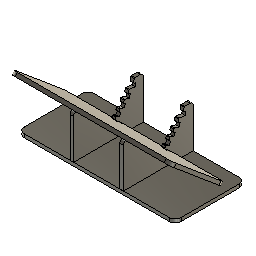
Stand1 (Autodesk Fusion 360 design; units mm, degrees)
Autodesk Fusion 360 part; units mm, degrees
sketch "スケッチ1" plane through (0, 0, 0) normal (0, 0, 1) x (1, 0, 0) in component "top1"
  line L0 (0, 0) -> (138, 0)
  line L1 (138, 0) -> (138, 60)
  line L2 (138, 60) -> (0, 60)
  line L3 (0, 60) -> (0, 0)
  line L4 (46.1, 60) -> (49, 60)
  line L5 (49, 60) -> (49, 54)
  line L6 (49, 54) -> (46.1, 54)
  line L7 (46.1, 54) -> (46.1, 60)
  line L8 (89, 60) -> (91.9, 60)
  line L9 (91.9, 60) -> (91.9, 54)
  line L10 (91.9, 54) -> (89, 54)
  line L11 (89, 54) -> (89, 60)
  line L12 (0, 60) -> (46.1, 54) construction
  line L13 (91.9, 54) -> (138, 60) construction
  line L14 (49, 54) -> (89, 54) construction
  dimension "d1" = 138
  dimension "d2" = 60
  dimension "d52" = 2.9
  dimension "d53" = 6
  dimension "d54" = 40
  constraint horizontal L0
  constraint vertical L1
  constraint horizontal L2
  constraint vertical L3
  constraint coincident L0.start L3.end
  constraint horizontal L4
  constraint vertical L5
  constraint horizontal L6
  constraint vertical L7
  constraint coincident L2 L4.start
  constraint horizontal L8
  constraint vertical L9
  constraint horizontal L10
  constraint vertical L11
  constraint coincident L2 L8.start
  constraint equal L5 L11
  constraint equal L6 L10
  constraint equal L12 L13
  measures "d1" distance of L0.start L0.end
  measures "d2" distance of L0.start L2.end
  measures "d52" distance of L5.end L6.end
  measures "d53" distance of L4.start L6.end
  measures "d54" distance of L5.end L10.end
extrude "押し出し1" add sketch "スケッチ1" along normal blind 3 contours L0 L1 L2 L3 L5 L6 L7 L9 L10 L11 makes body 1 in component "top1"
sketch "スケッチ1 (2)" plane through (0, 0, 0) normal (0, 0, 1) x (1, 0, 0) in component "base1"
  line L0 (-154.8575, 0.2102) -> (-19.8575, 0.2102)
  line L1 (-19.8575, 0.2102) -> (-19.8575, 60.2102)
  line L2 (-19.8575, 60.2102) -> (-154.8575, 60.2102)
  line L3 (-154.8575, 60.2102) -> (-154.8575, 0.2102)
  line L4 (-110.2575, 35.2102) -> (-107.3575, 35.2102)
  line L5 (-107.3575, 35.2102) -> (-107.3575, 25.2102)
  line L6 (-107.3575, 25.2102) -> (-110.2575, 25.2102)
  line L7 (-110.2575, 25.2102) -> (-110.2575, 35.2102)
  line L8 (-67.3575, 35.2102) -> (-64.4575, 35.2102)
  line L9 (-64.4575, 35.2102) -> (-64.4575, 25.2102)
  line L10 (-64.4575, 25.2102) -> (-67.3575, 25.2102)
  line L11 (-67.3575, 25.2102) -> (-67.3575, 35.2102)
  line L12 (-110.2575, 30.2102) -> (-154.8575, 30.2102) construction
  line L13 (-64.4575, 30.2102) -> (-19.8575, 30.2102) construction
  line L14 (-107.3575, 30.2102) -> (-67.3575, 30.2102) construction
  dimension "d5" = 135
  dimension "d6" = 60
  dimension "d45" = 10
  dimension "d46" = 2.9
  dimension "d47" = 40
  constraint horizontal L0
  constraint vertical L1
  constraint horizontal L2
  constraint vertical L3
  constraint horizontal L4
  constraint vertical L5
  constraint horizontal L6
  constraint vertical L7
  constraint horizontal L8
  constraint vertical L9
  constraint horizontal L10
  constraint vertical L11
  constraint equal L5 L11
  constraint equal L4 L8
  constraint midpoint L7 L12.start
  constraint midpoint L3 L12.end
  constraint midpoint L9 L13.start
  constraint midpoint L1 L13.end
  constraint midpoint L5 L14.start
  constraint midpoint L11 L14.end
  constraint horizontal L12
  constraint horizontal L14
  constraint equal L12 L13
  measures "d5" distance of L0.start L0.end
  measures "d6" distance of L0.start L2.end
  measures "d45" distance of L4.start L6.end
  measures "d46" distance of L4.start L4.end
  measures "d47" distance of L14.start L14.end
extrude "押し出し1'" add sketch "スケッチ1 (2)" along normal blind 3 separate body makes body 2 in component "base1"
sketch "スケッチ1 (3)" plane through (0, 0, 0) normal (1, 0, 0) x (0, 1, 0) in component "leg1"
  line L0 (82.5839, 7.0167) -> (142.5839, 7.0167)
  line L1 (142.5839, 7.0167) -> (142.5839, 43.8195)
  line L2 (142.5839, 43.8195) -> (82.5839, 43.8195)
  line L3 (82.5839, 43.8195) -> (82.5839, 7.0167)
  line L4 (116.2681, 18.4163) -> (82.5839, 46.6808)
  line L5 (107.5839, 7.0167) -> (117.5839, 7.0167)
  line L6 (117.5839, 7.0167) -> (117.5839, 4.1167)
  line L7 (117.5839, 4.1167) -> (107.5839, 4.1167)
  line L8 (107.5839, 4.1167) -> (107.5839, 7.0167)
  line L9 (112.5839, 4.1167) -> (112.5839, 7.0167) construction
  line L10 (83.1719, 45.4622) -> (119.7719, 22.592) construction
  line L11 (116.2681, 18.4163) -> (117.8002, 17.1308)
  line L12 (117.8002, 17.1308) -> (119.7286, 19.4289)
  line L13 (119.7286, 19.4289) -> (118.1965, 20.7145)
  line L14 (83.1268, 44.9274) -> (123.4494, 26.9747) construction
  line L15 (119.7719, 22.592) -> (121.8255, 21.3087)
  line L16 (121.8255, 21.3087) -> (123.4153, 23.8529)
  line L17 (123.4153, 23.8529) -> (121.7192, 24.9127)
  line L18 (82.9195, 44.5409) -> (127.47, 31.7662) construction
  line L19 (123.4494, 26.9747) -> (126.0624, 25.8113)
  line L20 (126.0624, 25.8113) -> (127.2826, 28.5519)
  line L21 (127.2826, 28.5519) -> (125.4555, 29.3654)
  line L22 (127.47, 31.7662) -> (130.6765, 30.8468)
  line L23 (116.2681, 18.4163) -> (137.5839, 43.8195)
  line L24 (82.5839, 44.1954) -> (132.0642, 37.2414) construction
  line L25 (132.0642, 37.2414) -> (135.9011, 36.7022)
  line L26 (135.9011, 36.7022) -> (136.3186, 39.673)
  line L27 (136.3186, 39.673) -> (134.3381, 39.9513)
  circle A0 centre (85.0839, 41.3195) radius 2.5
  line L28 (118.1965, 20.7145) -> (119.4826, 22.7727)
  line L29 (121.7192, 24.9127) -> (122.7716, 27.2764)
  line L30 (122.7716, 27.2764) -> (123.4494, 26.9747)
  line L31 (125.4555, 29.3654) -> (126.2447, 32.1176)
  line L32 (126.2447, 32.1176) -> (127.47, 31.7662)
  line L33 (130.146, 37.511) -> (132.0642, 37.2414)
  line L34 (134.3381, 39.9513) -> (134.8818, 43.8195)
  line L35 (119.4826, 22.7727) -> (119.7719, 22.592)
  line L36 (130.6765, 30.8468) -> (131.5034, 33.7306)
  line L37 (131.5034, 33.7306) -> (129.5809, 34.2818)
  line L38 (129.5809, 34.2818) -> (130.146, 37.511)
  dimension "d16" = 10
  dimension "d17" = 2.9
  dimension "d26" = 3
  dimension "d27" = 8
  dimension "d28" = 8
  dimension "d29" = 8
  dimension "d36" = 2
  dimension "d40" = 60
  dimension "d41" = 5
  dimension "d63" = 8
  dimension "d68" = 5
  dimension "d81" = 8
  constraint horizontal L0
  constraint vertical L1
  constraint horizontal L2
  constraint vertical L3
  constraint coincident L3 L24.start
  constraint horizontal L5
  constraint vertical L6
  constraint horizontal L7
  constraint vertical L8
  constraint coincident L0 L5.start
  constraint midpoint L7 L9.start
  constraint midpoint L0 L9.end
  constraint vertical L9
  constraint perpendicular L11 L12
  constraint perpendicular L10 L16
  constraint collinear L10 L15
  constraint equal L12 L16
  constraint perpendicular L19 L20
  constraint perpendicular L20 L21
  constraint collinear L14 L19
  constraint collinear L18 L22
  constraint equal L16 L20
  constraint coincident L10.end L23
  constraint coincident L13.end L23
  constraint coincident L17.end L23
  constraint coincident L14.end L23
  constraint coincident L21.end L23
  constraint coincident L18.end L23
  constraint equal L13 L17
  constraint equal L17 L21
  constraint perpendicular L4 L23
  constraint coincident L23.end L2
  constraint coincident L23 L24.end
  constraint perpendicular L25 L26
  constraint coincident L23 L27.end
  constraint perpendicular L26 L27
  constraint collinear L24 L25
  constraint collinear L4 L11
  constraint perpendicular L12 L13
  constraint perpendicular L16 L17
  constraint tangent L3 A0
  constraint tangent L2 A0
  constraint coincident L3 L4.end
  constraint tangent L4 A0
  constraint tangent L10 A0
  constraint tangent L14 A0
  constraint tangent L18 A0
  constraint tangent L24 A0
  constraint coincident L10 L28.end
  constraint perpendicular L10 L28
  constraint coincident L14 L29.end
  constraint perpendicular L14 L29
  constraint coincident L18 L31.end
  constraint perpendicular L18 L31
  constraint coincident L24 L33.start
  constraint coincident L2 L34.end
  constraint perpendicular L27 L34
  constraint perpendicular L22 L36
  constraint coincident L23 L37.end
  constraint perpendicular L36 L37
  constraint equal L20 L36
  constraint equal L26 L36
  constraint equal L21 L37
  constraint equal L27 L37
  measures "d16" distance of L5.start L5.end
  measures "d17" distance of L5.start L7.end
  measures "d26" distance of L11.end L12.end
  measures "d27" angle of L4 L10
  measures "d28" angle of L10 L14
  measures "d29" angle of L14 L18
  measures "d36" distance of L12.end L13.end
  measures "d40" distance of L0.start L0.end
  measures "d41" distance of L23.end L1.end
  measures "d63" angle of L2 L24
  measures "d68" diameter of A0
  measures "d81" angle of L18 L24
extrude "押し出し1''" add sketch "スケッチ1 (3)" along normal blind 3 separate body contours L0 L1 L2 L3 L4 L5 L11 L12 L13 L15 L16 L17 L19 L20 L21 L22 L23 L25 L26 L27 A0 L36 L37 | L0 L5 L6 L7 L8 | A0 | L2 L23 L34 | L23 L28 L35 | L23 L33 L38 | L23 L29 L30 | L23 L31 L32 makes body 3 in component "leg1"
fillet "フィレット1" radius 5 4 edges at (-154.8575, 0.2102, 1.5) (-19.8575, 0.2102, 1.5) (-154.8575, 60.2102, 1.5) (-19.8575, 60.2102, 1.5) on bodies 2 in component "base1"
fillet "フィレット1'" radius 5 4 edges at (0, 0, 1.5) (0, 60, 1.5) (138, 0, 1.5) (138, 60, 1.5) on bodies 1 in component "top1"
fillet "フィレット2" radius 2.5 1 edges at (1.5, 142.5839, 43.8195) on bodies 3 in component "leg1"
fillet "フィレット2" radius 0.5 10 edges at (1.5, 134.8818, 43.8195) (1.5, 134.3381, 39.9513) (1.5, 130.146, 37.511) (1.5, 129.5809, 34.2818) (1.5, 126.2447, 32.1176) (1.5, 125.4555, 29.3654) (1.5, 122.7716, 27.2764) (1.5, 121.7192, 24.9127) (1.5, 119.4826, 22.7727) (1.5, 118.1965, 20.7145) on bodies 3 in component "leg1"
component "top1" placed x (1, 0, 0) y (0, 0.766044, -0.642788) z (0, 0.642788, 0.766044) at (-156.4075, -5.9399, 47.7246)
component "base1" placed x (1, 0, 0) y (0, 1, 0) z (0, 0, 1) at (0, 0, 0)
component "leg1" placed x (1, 0, 0) y (0, 1, 0) z (0, 0, 1) at (-67.4575, -82.3737, -4.1167)
component "leg1" placed x (1, 0, 0) y (0, 1, 0) z (0, 0, 1) at (-110.3575, -82.3737, -4.1167)
equation "d17 = d46"
equation "d27 = d63"
equation "d28 = d63"
equation "d29 = d63"
equation "d40 = d2"
equation "d46 = d52"
equation "d47 = d54"
equation "d81 = d63"
